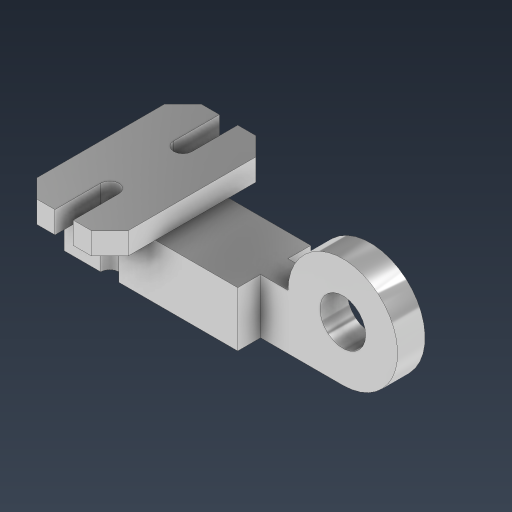
# Autodesk Inventor part: Peça1
Saved by Autodesk Inventor 2024 (Build 280153000, 153)
## iProperties
Created: 2024-02-09
Part Number: Peça1
Material: Alumínio 6061
Document SubType Name: Modeling
Designer: Administrator
Density: 2.7 g/cm^3
Appearance: Cromado - Polido
Author: Administrator
Autodesk Inventor part; units mm, degrees
ref_plane "YZ Plane" through (0, 0, 0) normal (1, 0, 0) x (0, 1, 0)
ref_plane "XZ Plane" through (0, 0, 0) normal (0, 1, 0) x (-1, 0, 0)
ref_plane "XY Plane" through (0, 0, 0) normal (0, 0, 1) x (1, 0, 0)
sketch "Esboço1" plane through (0, 0, 0) normal (0, 0, 1) x (1, 0, 0)
  line L0 (0, 0) -> (95, 0)
  line L1 (95, 0) -> (95, 30)
  line L2 (95, 30) -> (0, 30)
  line L3 (0, 30) -> (0, 0)
  line L4 (0, 30) -> (50, 30)
  line L5 (50, 30) -> (50, 42)
  line L6 (50, 42) -> (0, 42)
  line L7 (0, 42) -> (0, 30)
  line L8 (95, 0) -> (140, 0)
  line L9 (110, 30) -> (95, 30)
  line L10 (95, 30) -> (95, 0)
  arc A0 (140, 0) -> (110, 30) centre (140, 30) ccw
  circle A1 centre (140, 30) radius 12.5
  point P0 (0, 15)
  dimension "d0" = 95
  dimension "d1" = 30
  dimension "d3" = 50
  dimension "d4" = 12
  dimension "d5" = 30
  dimension "d6" = 140
  dimension "d7" = 25
  constraints: 22 end point, 5 parallel, 3 horizontal, 2 centre point, 2 perpendicular, 2 point on circle, 1 coincident, 1 collinear, 1 midpoint, 1 tangent
  measures "d0" distance from line of L1 point (0, 15)
  measures "d1" distance between parallel lines of L0 L2
  measures "d3" distance between parallel lines of L7 L5
  measures "d4" distance between parallel lines of L2 L6
  measures "d5" radius of A0
  measures "d6" distance from line of A0.centre L3
  measures "d7" diameter of A1
extrude "Extrusão1" add sketch "Esboço1" along normal mid plane 90 contours L7 L6 L5 L2
extrude "Extrusão2" add sketch "Esboço1" along normal mid plane 15 contours L1 L9 A0 L8
extrude "Extrusão3" add sketch "Esboço1" along normal mid plane 40 contours L3 L2 L1 L0
sketch "Esboço2" plane through (0, 42, 45) normal (0, 1, 0) x (1, 0, 0)
  line L0 (25, 115) -> (25, 65) construction
  line L1 (50, 90) -> (0, 90) projected
  line L2 (20, 115) -> (20, 65)
  line L3 (30, 65) -> (30, 115)
  arc A0 (30, 115) -> (20, 115) centre (25, 115) ccw
  arc A1 (20, 65) -> (30, 65) centre (25, 65) ccw
  line L4 (25, -25) -> (25, 25) construction
  line L5 (0, 0) -> (50, 0) projected
  line L6 (20, -25) -> (20, 25)
  line L7 (30, 25) -> (30, -25)
  arc A2 (20, -25) -> (30, -25) centre (25, -25) ccw
  arc A3 (30, 25) -> (20, 25) centre (25, 25) ccw
  point P0 (0, 45)
  point P1 (25, 90)
  point P2 (25, 0)
  point P3 (20, 0)
  point P4 (30, 0)
  point P5 (30, 90)
  point P6 (20, 90)
  dimension "d14" = 5
  dimension "d15" = 5
  dimension "d16" = 25
  dimension "d17" = 25
  constraints: 16 end point, 8 point on circle, 8 tangent, 4 centre point, 4 midpoint, 2 parallel, 1 perpendicular, 1 point on line
  measures "d14" radius of A1
  measures "d15" radius of A3
  measures "d16" distance from line of L0.end L1
  measures "d17" distance from line of L4.end L5
extrude "Extrusão4" cut sketch "Esboço2" against normal through all contours L6 A3 L7 L5
extrude "Extrusão5" cut sketch "Esboço2" against normal through all contours L3 A1 L2 L1
chamfer "Chanfro1" distance 10 angle 45 4 edges at (0, 36, 45) (50, 36, 45) (50, 36, -45) (0, 36, -45)
